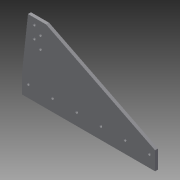
# Autodesk Inventor part: rail mounting bracket
Saved by Autodesk Inventor 2015 SP1 (Build 190203100, 203)
## iProperties
Created: 2015-01-15
Part Number: rail mounting bracket
Material: Generic
Document SubType Name: Modeling
Designer: Jarod
Density: 1 g/cm^3
Appearance: Default
Author: Jarod
Autodesk Inventor part; units mm, degrees
ref_plane "YZ Plane" through (0, 0, 0) normal (1, 0, 0) x (0, 1, 0)
ref_plane "XZ Plane" through (0, 0, 0) normal (0, 1, 0) x (-1, 0, 0)
ref_plane "XY Plane" through (0, 0, 0) normal (0, 0, 1) x (1, 0, 0)
sketch "Sketch1" plane through (0, 0, 0) normal (0, 0, 1) x (1, 0, 0)
  line L0 (0, 0) -> (190.5, 0) construction
  line L1 (190.5, 0) -> (190.5, 152.4) construction
  line L2 (190.5, 152.4) -> (0, 152.4) construction
  line L3 (0, 152.4) -> (0, 0) construction
  line L4 (0, 0) -> (190.5, 0)
  line L5 (0, 0) -> (0, 38.1)
  line L6 (0, 0) -> (38.1, 0) construction
  line L7 (190.5, 0) -> (190.5, 38.1)
  line L8 (190.5, 0) -> (228.6, 0) construction
  line L9 (190.5, 152.4) -> (57.15, 152.4) construction
  line L10 (190.5, 152.4) -> (323.85, 152.4) construction
  line L11 (57.15, 152.4) -> (19.05, 152.4) construction
  line L12 (0, 38.1) -> (19.05, 152.4)
  line L13 (19.05, 152.4) -> (57.15, 152.4)
  line L14 (57.15, 152.4) -> (190.5, 38.1)
  circle A0 centre (12.7, 25.4) radius 3.175
  circle A1 centre (63.5, 25.4) radius 3.175
  circle A2 centre (31.75, 139.7) radius 3.175
  circle A3 centre (44.45, 127) radius 3.175
  circle A4 centre (31.75, 114.3) radius 3.175
  circle A5 centre (44.45, 101.6) radius 3.175
  circle A6 centre (114.3, 25.4) radius 3.175
  circle A7 centre (165.1, 25.4) radius 3.175
  dimension "d0" = 190.5
  dimension "d1" = 152.4
  dimension "d2" = 12.7
  dimension "d3" = 50.8
  dimension "d8" = 25.4
  dimension "d9" = 25.4
  dimension "d10" = 38.1
  dimension "d11" = 90
  dimension "d12" = 38.1
  dimension "d13" = 90
  dimension "d14" = 133.35
  dimension "d15" = 180
  dimension "d16" = 38.1
  dimension "d17" = 12.7
  dimension "d18" = 12.7
  dimension "d19" = 12.7
  dimension "d20" = 12.7
  dimension "d21" = 12.7
  dimension "d22" = 25.4
  dimension "d23" = 38.1
  dimension "d24" = 50.8
  dimension "d25" = 6.35
  dimension "d26" = 6.35
  dimension "d29" = 6.35
  dimension "d30" = 6.35
  dimension "d31" = 6.35
  dimension "d32" = 6.35
  dimension "d35" = 50.8
  dimension "d36" = 50.8
  dimension "d38" = 6.35
  dimension "d39" = 6.35
  dimension "d46" = 25.4
  dimension "d47" = 25.4
  constraints: 30 end point, 8 centre point, 8 coincident, 6 horizontal, 3 collinear, 3 equal length, 2 parallel, 1 perpendicular, 1 point on line
  measures "d0" distance of L2.end L1.end
  measures "d1" distance of L1.end L0.end
  measures "d2" distance from line of point (12.7, 25.4) L3
  measures "d3" distance of point (63.5, 25.4) point (12.7, 25.4)
  measures "d8" distance from line of L0 point (63.5, 25.4)
  measures "d9" distance from line of L0 point (12.7, 25.4)
  measures "d10" distance of L0.start L5.end
  measures "d11" angle of L6 L5
  measures "d12" distance of L0.end L7.end
  measures "d13" angle of L8 L7
  measures "d14" distance of L1.end L9.end
  measures "d15" angle of L9 L10
  measures "d16" distance of L9.end L11.end
  measures "d17" horizontal distance of point (31.75, 139.7) L11.end
  measures "d18" horizontal distance of point (44.45, 127) L9.end
  measures "d19" horizontal distance of L11.end point (31.75, 114.3)
  measures "d20" horizontal distance of L9.end point (44.45, 101.6)
  measures "d21" distance from line of L11 point (31.75, 139.7)
  measures "d22" distance from line of L2 point (44.45, 127)
  measures "d23" distance from line of L11 point (31.75, 114.3)
  measures "d24" distance from line of point (44.45, 101.6) L11
  measures "d25" diameter of A0
  measures "d26" diameter of A1
  measures "d29" diameter of A2
  measures "d30" diameter of A3
  measures "d31" diameter of A4
  measures "d32" diameter of A5
  measures "d35" distance of point (114.3, 25.4) point (63.5, 25.4)
  measures "d36" distance of point (165.1, 25.4) point (114.3, 25.4)
  measures "d38" diameter of A6
  measures "d39" diameter of A7
  measures "d46" distance from line of L0 point (114.3, 25.4)
  measures "d47" distance from line of L0 point (165.1, 25.4)
extrude "Extrusion4" add sketch "Sketch1" along normal blind 6.35
sketch "Sketch3" plane through (0, 0, 6.35) normal (0, 0, 1) x (1, 0, 0)
  line L0 (0, 0) -> (0, 25.4)
  line L1 (0, 38.1) -> (0, 0) projected
  line L2 (0, 0) -> (12.7, 0)
  line L3 (0, 0) -> (190.5, 0) projected
  line L4 (0, 25.4) -> (12.7, 0)
  dimension "d50" = 25.4
  dimension "d51" = 12.7
  constraints: 6 end point, 2 point on line
  measures "d50" distance of L0.start L0.end
  measures "d51" distance of L0.start L2.end
extrude "Extrusion5" cut sketch "Sketch3" against normal blind 6.35
sketch "Sketch4" plane through (0, 0, 6.35) normal (0, 0, 1) x (1, 0, 0)
  line L0 (0, 38.1) -> (0, 25.4) projected
  line L1 (12.7, 0) -> (190.5, 0) projected
  circle A0 centre (28.575, 52.3875) radius 3.175
  circle A1 centre (44.45, 52.3875) radius 3.175
  circle A2 centre (38.1, 69.85) radius 4.7625
  point P0 (0, 0)
  dimension "d54" = 28.575
  dimension "d55" = 44.45
  dimension "d56" = 52.3875
  dimension "d57" = 52.3875
  dimension "d58" = 69.85
  dimension "d59" = 38.1
  dimension "d60" = 6.35
  dimension "d61" = 6.35
  dimension "d62" = 9.525
  constraints: 3 centre point, 3 coincident
  measures "d54" distance from line of point (28.575, 52.388) L0
  measures "d55" distance from line of point (44.45, 52.388) L0
  measures "d56" distance from line of L1 point (28.575, 52.388)
  measures "d57" distance from line of L1 point (44.45, 52.388)
  measures "d58" distance from line of L1 point (38.1, 69.85)
  measures "d59" distance from line of L0 point (38.1, 69.85)
  measures "d60" diameter of A0
  measures "d61" diameter of A1
  measures "d62" diameter of A2
extrude "Extrusion6" cut sketch "Sketch4" against normal blind 6.35
body "Solid3"
